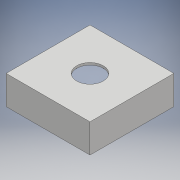
# Autodesk Inventor part: lupa_camera_mount
Saved by Autodesk Inventor 2018 (Build 220112000, 112)
## iProperties
Created: 2018-01-19
Part Number: lupa_camera_mount
Material: Generic
Document SubType Name: Modeling
Designer: matth
Density: 1 g/cm^3
Appearance: Default
Author: matth
Autodesk Inventor part; units mm, degrees
ref_plane "YZ Plane" through (0, 0, 0) normal (1, 0, 0) x (0, 1, 0)
ref_plane "XZ Plane" through (0, 0, 0) normal (0, 1, 0) x (-1, 0, 0)
ref_plane "XY Plane" through (0, 0, 0) normal (0, 0, 1) x (1, 0, 0)
sketch "Sketch1" plane through (0, 0, 0) normal (0, 0, 1) x (1, 0, 0)
  line L0 (-12.2234, 6.6825) -> (23.6766, 6.6825)
  line L1 (23.6766, 6.6825) -> (23.6766, -29.2175)
  line L2 (23.6766, -29.2175) -> (-12.2234, -29.2175)
  line L3 (-12.2234, -29.2175) -> (-12.2234, 6.6825)
  line L4 (-13.2234, 7.6825) -> (24.6766, 7.6825)
  line L5 (24.6766, 7.6825) -> (24.6766, -30.2175)
  line L6 (24.6766, -30.2175) -> (-13.2234, -30.2175)
  line L7 (-13.2234, -30.2175) -> (-13.2234, 7.6825)
  point P0 (0, 0)
  dimension "d0" = 35.9
  dimension "d1" = 35.9
  dimension "d2" = 37.9
  dimension "d3" = 37.9
  dimension "d4" = 1
  dimension "d5" = 1
  constraints: 16 end point, 4 parallel, 2 horizontal, 2 perpendicular
  measures "d0" distance of L1.end L2.end
  measures "d1" distance of L0.end L1.end
  measures "d2" distance of L5.end L6.end
  measures "d3" distance of L4.end L5.end
  measures "d4" distance between parallel lines of L4 L0
  measures "d5" distance between parallel lines of L7 L3
extrude "Extrusion1" add sketch "Sketch1" along normal blind 12
sketch "Sketch2" plane through (0, 0, 12) normal (0, 0, 1) x (1, 0, 0)
  line L0 (-13.2234, -30.2175) -> (-13.2234, 7.6825) projected
  line L1 (-13.2234, -30.2175) -> (24.6766, -30.2175) projected
  line L2 (-13.2234, 7.6825) -> (24.6766, 7.6825)
  line L3 (24.6766, 7.6825) -> (24.6766, -30.2175)
  line L4 (24.6766, -30.2175) -> (-13.2234, -30.2175)
  line L5 (-13.2234, -30.2175) -> (-13.2234, 7.6825)
  point P0 (0, 0)
  constraints: 8 end point, 2 parallel, 1 horizontal, 1 perpendicular
extrude "Extrusion2" add sketch "Sketch2" along normal blind 1
sketch "Sketch3" plane through (0, 0, 13) normal (0, 0, 1) x (1, 0, 0)
  circle A0 centre (5.7266, -11.2675) radius 6
  line L0 (-13.2234, 7.6825) -> (-13.2234, -30.2175) projected
  line L1 (-13.2234, -30.2175) -> (24.6766, -30.2175) projected
  point P0 (0, 0)
  dimension "d10" = 12
  dimension "d11" = 18.95
  dimension "d12" = 18.95
  dimension "d13" = 37.9
  constraints: 1 centre point
  measures "d10" diameter of A0
  measures "d11" distance from line of L0 A0.centre
  measures "d12" distance from line of L1 A0.centre
  measures "d13" distance of L0.start L0.end
extrude "Extrusion3" cut sketch "Sketch3" against normal blind 1
equation "\"d11\" = 0.5 * d13"
equation "\"d12\" = 0.5 * d13"
body "Solid1"
